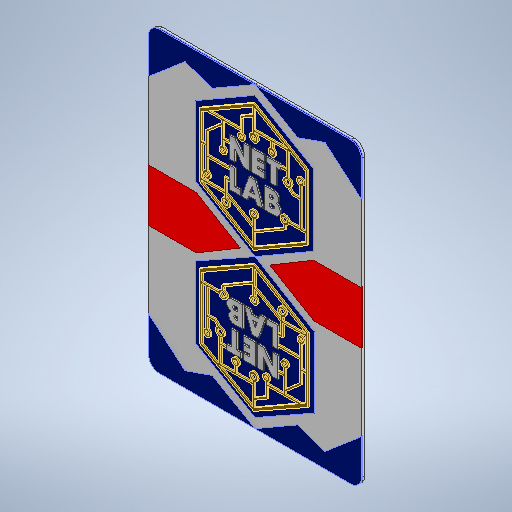
# Autodesk Inventor part: 4ofethernet
Saved by Autodesk Inventor 2025 (Build 290162010, 162A)
## iProperties
Created: 2024-07-12
Part Number: 4ofethernet
Material: Generic
Document SubType Name: Modeling
Designer: joshu
Density: 1 g/cm^3
Appearance: Default
Author: joshu
Autodesk Inventor part; units mm, degrees
(part 1 of 2)
ref_plane "YZ Plane" through (0, 0, 0) normal (1, 0, 0) x (0, 1, 0)
ref_plane "XZ Plane" through (0, 0, 0) normal (0, 1, 0) x (-1, 0, 0)
ref_plane "XY Plane" through (0, 0, 0) normal (0, 0, 1) x (1, 0, 0)
sketch "Sketch1" plane through (0, 0, 0) normal (0, 0, 1) x (1, 0, 0)
  line L0 (0, 0) -> (63.5, 0)
  line L1 (63.5, 0) -> (63.5, 88.9)
  line L2 (63.5, 88.9) -> (0, 88.9)
  line L3 (0, 88.9) -> (0, 0)
  line L4 (31.75, 44.45) -> (49.3079, 54.587)
  line L5 (49.3079, 54.587) -> (49.3079, 75.7826)
  line L6 (49.3079, 75.7826) -> (31.6801, 86.0828)
  line L7 (31.6801, 86.0828) -> (13.967, 75.8563)
  line L8 (13.967, 75.8563) -> (13.967, 55.04)
  line L9 (13.967, 55.04) -> (31.75, 44.45)
  line L10 (15.5263, 74.956) -> (31.6754, 84.2796)
  line L11 (31.6754, 84.2796) -> (47.7487, 74.8877)
  line L12 (47.7487, 74.8877) -> (47.7487, 55.4872)
  line L13 (47.7487, 55.4872) -> (31.7622, 46.2575)
  line L14 (31.7622, 46.2575) -> (15.5263, 55.9263)
  line L15 (15.5263, 55.9263) -> (15.5263, 74.956)
  line L16 (47.1273, 56.0392) -> (31.9379, 47.2671)
  line L17 (31.3664, 47.317) -> (16.2977, 56.192)
  line L18 (41.8086, 77.4972) -> (32.0418, 77.4972)
  line L19 (42.0908, 76.9257) -> (42.0908, 70.0939)
  line L20 (41.5193, 72.1376) -> (39.6994, 72.1376)
  line L21 (39.6994, 72.1376) -> (39.6994, 71.5661)
  line L22 (39.6994, 71.5661) -> (41.5193, 71.5661)
  arc A0 (31.465, 76.5861) -> (32.0365, 76.5861) centre (31.7507, 75.3324) ccw
  arc A1 (36.8763, 75.3571) -> (37.4478, 75.3571) centre (37.162, 74.2504) ccw
  circle A2 centre (37.162, 74.2504) radius 0.4762
  circle A3 centre (31.7507, 75.3324) radius 0.6191
  line L23 (45.9318, 69.8545) -> (45.9318, 58.9507)
  line L24 (45.3603, 66.7769) -> (43.3841, 66.7769)
  line L25 (43.1915, 66.2054) -> (45.3603, 66.2054)
  circle A4 centre (41.805, 68.7917) radius 0.762
  line L26 (43.1915, 66.2054) -> (41.9826, 67.4703)
  line L27 (43.3841, 66.7769) -> (42.5287, 67.6719)
  arc A5 (45.9318, 69.8545) -> (45.3603, 69.8545) centre (45.646, 70.9598) ccw
  circle A6 centre (45.646, 70.9598) radius 0.5715
  line L28 (40.6132, 56.5528) -> (40.6132, 57.4113)
  circle A7 centre (40.899, 58.665) radius 0.7144
  line L29 (32.0418, 83.1688) -> (32.0418, 77.4972)
  line L30 (32.0365, 76.9257) -> (32.0365, 76.5861)
  line L31 (32.0365, 76.9257) -> (36.8763, 76.9257)
  line L32 (36.8763, 75.3571) -> (36.8763, 76.9257)
  line L33 (37.4478, 76.9257) -> (37.4478, 75.3571)
  line L34 (37.4478, 76.9257) -> (41.5193, 76.9257)
  line L35 (42.0908, 76.9257) -> (42.7928, 76.9257)
  line L36 (32.0365, 83.1719) -> (41.8086, 77.4972)
  line L37 (42.7928, 76.9257) -> (47.1273, 74.4086)
  line L38 (41.5193, 70.0939) -> (41.5193, 71.5661)
  line L39 (41.5193, 72.1376) -> (41.5193, 76.9257)
  arc A8 (41.5193, 70.0939) -> (41.9826, 67.4703) centre (41.805, 68.7917) ccw
  arc A9 (42.5287, 67.6719) -> (42.0908, 70.0939) centre (41.805, 68.7917) ccw
  line L40 (45.3603, 58.9507) -> (45.3603, 66.2054)
  line L41 (45.3603, 66.7769) -> (45.3603, 69.8545)
  line L42 (47.1273, 58.9507) -> (45.9318, 58.9507)
  line L43 (45.3603, 58.9507) -> (42.1527, 58.9507)
  line L44 (42.1475, 58.3804) -> (47.1273, 58.3804)
  line L45 (41.1819, 57.4161) -> (41.1819, 56.2658)
  arc A10 (42.1527, 58.9507) -> (40.6132, 57.4113) centre (40.899, 58.665) ccw
  arc A11 (41.1819, 57.4161) -> (42.1475, 58.3804) centre (40.899, 58.665) ccw
  line L46 (47.1273, 74.4086) -> (47.1273, 58.9507)
  line L47 (47.1273, 58.3804) -> (47.1273, 56.0392)
  line L48 (27.6974, 78.6822) -> (27.6974, 79.0777)
  line L49 (28.2689, 78.6822) -> (31.465, 80.528)
  line L50 (27.6974, 79.0777) -> (31.465, 81.2535)
  line L51 (31.465, 76.5861) -> (31.465, 80.528)
  line L52 (31.465, 81.2535) -> (31.465, 83.1596)
  line L53 (31.9379, 51.4601) -> (40.6132, 56.5528)
  line L54 (31.9379, 50.8392) -> (41.1819, 56.2658)
  line L55 (16.2977, 57.1448) -> (22.9994, 57.1448)
  line L56 (22.9994, 56.5733) -> (16.2977, 56.5733)
  line L57 (16.2977, 56.5733) -> (16.2977, 57.1448)
  line L58 (22.9994, 60.9472) -> (23.5709, 60.9472)
  line L59 (22.9994, 60.9472) -> (24.4329, 60.9472)
  line L60 (24.4329, 60.9472) -> (24.4329, 60.3757)
  line L61 (24.4329, 60.3757) -> (23.5709, 60.3757)
  line L62 (22.9994, 60.3757) -> (22.9994, 60.9472)
  line L63 (23.5709, 56.4373) -> (31.3664, 51.9861)
  line L64 (31.3664, 52.5972) -> (23.5709, 57.0484)
  arc A12 (31.9379, 54.3552) -> (31.3664, 54.3552) centre (31.6521, 55.5111) ccw
  circle A13 centre (31.6521, 55.5111) radius 0.6191
  arc A14 (22.9994, 55.5805) -> (23.5709, 55.5805) centre (23.2852, 54.3309) ccw
  circle A15 centre (23.2852, 54.3309) radius 0.7144
  line L65 (23.5709, 60.3757) -> (23.5709, 57.0484)
  line L66 (23.5709, 56.4373) -> (23.5709, 55.5805)
  line L67 (22.9994, 55.5805) -> (22.9994, 56.5733)
  line L68 (22.9994, 57.1448) -> (22.9994, 60.9472)
  line L69 (31.3664, 54.3552) -> (31.3664, 52.5972)
  line L70 (31.3664, 51.9861) -> (31.3664, 47.317)
  line L71 (31.9379, 47.2671) -> (31.9379, 50.8392)
  line L72 (31.9379, 51.4601) -> (31.9379, 54.3552)
  arc A16 (27.6974, 74.6924) -> (28.2689, 74.6924) centre (27.9831, 73.6844) ccw
  circle A17 centre (27.9831, 73.6844) radius 0.4763
  line L73 (18.5492, 75.7007) -> (27.6974, 75.7007)
  line L74 (22.769, 70.6818) -> (24.4329, 70.6818)
  line L75 (24.4329, 70.6818) -> (24.4329, 70.1103)
  line L76 (24.4329, 70.1103) -> (22.769, 70.1103)
  line L77 (22.769, 70.1103) -> (22.769, 70.2009)
  line L78 (16.2977, 66.7769) -> (17.4065, 66.7769)
  line L79 (17.978, 66.7769) -> (17.978, 66.2054)
  line L80 (17.4065, 66.2054) -> (16.2977, 66.2054)
  line L81 (17.978, 63.9706) -> (24.4329, 63.9706)
  line L82 (24.4329, 63.9706) -> (24.4329, 63.3991)
  line L83 (24.4329, 63.3991) -> (17.978, 63.3991)
  line L84 (17.4065, 66.7769) -> (17.4065, 70.2549)
  line L85 (17.978, 70.0307) -> (17.978, 66.7769)
  line L86 (17.4065, 70.2549) -> (22.1975, 74.4365)
  line L87 (17.978, 70.0307) -> (22.1975, 73.7135)
  arc A18 (22.1975, 68.5281) -> (22.769, 68.5281) centre (22.4833, 67.4703) ccw
  circle A19 centre (22.4833, 67.4703) radius 0.5239
  line L88 (16.2977, 74.4004) -> (17.5596, 75.1292)
  line L89 (18.5492, 75.7007) -> (31.465, 83.1596)
  line L90 (27.6974, 75.1292) -> (22.769, 75.1292)
  line L91 (22.1975, 75.1292) -> (17.5596, 75.1292)
  line L92 (22.1975, 74.4365) -> (22.1975, 75.1292)
  line L93 (28.2689, 74.6924) -> (28.2689, 78.6822)
  line L94 (22.769, 75.1292) -> (22.769, 70.6818)
  line L95 (22.769, 70.1103) -> (22.769, 68.5281)
  line L96 (22.1975, 67.8875) -> (22.1975, 67.9094)
  line L97 (22.1975, 68.5281) -> (22.1975, 73.7135)
  line L98 (16.2977, 56.192) -> (16.2977, 66.2054)
  line L99 (16.2977, 66.7769) -> (16.2977, 74.4004)
  line L100 (17.978, 63.9706) -> (17.978, 66.2054)
  line L101 (27.6974, 78.6822) -> (27.6974, 75.7007)
  line L102 (27.6974, 75.1292) -> (27.6974, 74.6924)
  line L103 (24.4329, 66.1976) -> (26.1474, 66.1976)
  line L104 (26.1474, 66.1976) -> (26.1474, 69.7075)
  line L105 (26.1474, 72.4542) -> (24.4329, 72.4542)
  line L106 (24.4329, 72.4542) -> (24.4329, 66.1976)
  line L107 (28.7777, 72.4542) -> (30.4922, 72.4542)
  line L108 (30.4922, 72.4542) -> (30.4922, 66.1976)
  line L109 (30.4922, 66.1976) -> (28.7777, 66.1976)
  line L110 (28.7777, 68.9443) -> (28.7777, 72.4542)
  line L111 (28.7777, 66.1976) -> (26.1474, 69.7075)
  line L112 (26.1474, 72.4542) -> (28.7777, 68.9443)
  line L113 (31.2537, 72.4542) -> (32.9682, 72.4542)
  line L114 (32.9682, 66.1976) -> (31.2537, 66.1976)
  line L115 (31.2537, 66.1976) -> (31.2537, 72.4542)
  line L116 (31.2537, 72.4542) -> (34.8385, 72.4542)
  line L117 (34.8385, 72.4542) -> (34.8385, 70.7397)
  line L118 (34.8385, 70.7397) -> (32.9682, 70.7397)
  line L119 (31.2537, 70.7397) -> (31.2537, 72.4542)
  line L120 (32.9682, 70.0633) -> (34.8385, 70.0633)
  line L121 (34.8385, 70.0633) -> (34.8385, 68.5393)
  line L122 (34.8385, 68.5393) -> (32.9682, 68.5393)
  line L123 (31.2537, 68.5393) -> (31.2537, 70.0633)
  line L124 (31.2537, 66.1976) -> (34.8385, 66.1976)
  line L125 (34.8385, 66.1976) -> (34.8385, 67.9121)
  line L126 (34.8385, 67.9121) -> (32.9682, 67.9121)
  line L127 (31.2537, 67.9121) -> (31.2537, 66.1976)
  line L128 (32.9682, 70.7397) -> (32.9682, 70.0633)
  line L129 (32.9682, 68.5393) -> (32.9682, 67.9121)
  line L130 (39.6994, 72.4422) -> (35.4849, 72.4422)
  line L131 (35.4849, 72.4422) -> (35.4849, 70.9182)
  line L132 (39.6994, 70.9182) -> (39.6994, 72.4422)
  line L133 (38.4466, 70.9182) -> (38.4466, 66.1976)
  line L134 (38.4466, 66.1976) -> (36.7321, 66.1976)
  line L135 (36.7321, 66.1976) -> (36.7321, 70.9182)
  line L136 (36.7321, 70.9182) -> (36.8763, 70.9182)
  line L137 (35.4849, 70.9182) -> (36.7321, 70.9182)
  line L138 (38.4466, 70.9182) -> (39.6994, 70.9182)
  line L139 (24.4329, 64.6461) -> (26.1474, 64.6461)
  line L140 (26.1474, 64.6461) -> (26.1474, 59.9044)
  line L141 (26.1474, 58.3804) -> (24.4329, 58.3804)
  line L142 (24.4329, 58.3804) -> (24.4329, 64.6461)
  line L143 (24.4329, 58.3804) -> (27.8234, 58.3804)
  line L144 (27.8234, 58.3804) -> (27.8234, 59.9044)
  line L145 (27.8234, 59.9044) -> (26.1474, 59.9044)
  line L146 (24.4329, 59.9044) -> (24.4329, 58.3804)
  line L147 (28.1466, 58.3804) -> (29.8611, 58.3804)
  line L148 (29.8611, 58.3804) -> (30.3254, 59.5144)
  line L149 (30.3254, 59.5144) -> (32.2304, 59.5144)
  line L150 (30.3254, 64.6461) -> (32.2304, 64.6461)
  line L151 (28.1466, 58.3804) -> (30.3254, 64.6461)
  line L152 (32.728, 58.3804) -> (34.4425, 58.3804)
  line L153 (32.728, 58.3804) -> (32.2304, 59.5144)
  line L154 (34.4425, 58.3804) -> (32.2304, 64.6461)
  line L155 (30.6203, 60.8236) -> (31.9379, 60.8236)
  line L156 (31.9379, 60.8236) -> (31.2779, 62.4085)
  line L157 (31.2779, 62.4085) -> (30.6203, 60.8236)
  line L158 (34.9216, 58.3804) -> (34.9216, 64.6461)
  line L159 (34.9216, 64.6461) -> (37.8691, 64.6461)
  line L160 (34.9216, 58.3804) -> (37.8691, 58.3804)
  line L161 (36.5599, 59.8143) -> (36.5599, 60.939)
  line L162 (36.5599, 62.1736) -> (36.5599, 63.1944)
  line L163 (36.5599, 63.1944) -> (37.2133, 63.1944)
  line L164 (36.5599, 62.1736) -> (37.2133, 62.1736)
  arc A20 (37.2133, 62.1736) -> (37.2133, 63.1944) centre (37.055, 62.684) ccw
  line L165 (36.5599, 60.939) -> (37.4519, 60.939)
  line L166 (36.5599, 59.8143) -> (37.4396, 59.8143)
  arc A21 (37.4396, 59.8143) -> (37.4519, 60.939) centre (37.3959, 60.3772) ccw
  arc A22 (38.5631, 61.7817) -> (37.8691, 64.6461) centre (37.5266, 63.0469) ccw
  arc A23 (37.8691, 58.3804) -> (38.5631, 61.7817) centre (37.9604, 60.1332) ccw
  arc A24 (17.4065, 59.8724) -> (17.978, 59.8724) centre (17.6923, 58.815) ccw
  circle A25 centre (17.6923, 58.815) radius 0.5239
  line L167 (17.4065, 66.2054) -> (17.4065, 59.8724)
  line L168 (17.978, 59.8724) -> (17.978, 63.3991)
  line L169 (32.0418, 83.1688) -> (41.8086, 77.4972)
  line L170 (32.0418, 77.4972) -> (41.8086, 77.4972)
  line L171 (32.0418, 77.4972) -> (32.0418, 83.1688)
  line L172 (0, 44.45) -> (63.5, 44.45) construction
  line L173 (31.75, 88.9) -> (31.75, 0) construction
  line L174 (0, 52.2573) -> (14.2102, 52.2573)
  line L175 (14.2102, 52.2573) -> (27.3204, 44.45)
  line L176 (0, 36.6427) -> (14.2102, 36.6427)
  line L177 (14.2102, 36.6427) -> (27.3204, 44.45)
  line L178 (63.5, 52.2573) -> (49.2898, 52.2573)
  line L179 (49.2898, 52.2573) -> (36.1796, 44.45)
  line L180 (49.2898, 36.6427) -> (36.1796, 44.45)
  line L181 (63.5, 36.6427) -> (49.2898, 36.6427)
  line L182 (0, 75.0796) -> (10.8905, 84.3747)
  line L183 (10.8905, 84.3747) -> (18.9583, 81.5148)
  line L184 (18.9583, 81.5148) -> (31.75, 88.9)
  line L185 (63.5, 75.0796) -> (52.6095, 84.3747)
  line L186 (52.6095, 84.3747) -> (44.5417, 81.5148)
  line L187 (44.5417, 81.5148) -> (31.75, 88.9)
  line L188 (46.0393, 22.6946) -> (47.1481, 22.6946)
  line L189 (45.4678, 22.1231) -> (45.4678, 22.6946)
  line L190 (45.4678, 24.9294) -> (45.4678, 22.6946)
  line L191 (47.1481, 22.1231) -> (46.0393, 22.1231)
  line L192 (47.1481, 32.3267) -> (47.1481, 31.7552)
  line L193 (47.1481, 32.708) -> (47.1481, 22.6946)
  line L194 (47.1481, 31.7552) -> (40.4464, 31.7552)
  line L195 (40.4464, 32.3267) -> (47.1481, 32.3267)
  line L196 (45.4678, 29.0276) -> (45.4678, 25.5009)
  line L197 (46.0393, 22.6946) -> (46.0393, 29.0276)
  circle A26 centre (45.7535, 30.085) radius 0.5239
  arc A27 (46.0393, 29.0276) -> (45.4678, 29.0276) centre (45.7535, 30.085) ccw
  line L198 (20.6531, 11.9743) -> (16.3185, 14.4914)
  line L199 (21.355, 11.9743) -> (20.6531, 11.9743)
  line L200 (21.9265, 16.7624) -> (21.9265, 11.9743)
  line L201 (21.355, 11.9743) -> (21.355, 18.8061)
  line L202 (21.9265, 16.7624) -> (23.7464, 16.7624)
  line L203 (23.7464, 17.3339) -> (21.9265, 17.3339)
  line L204 (25.998, 11.9743) -> (21.9265, 11.9743)
  line L205 (26.5695, 13.5429) -> (26.5695, 11.9743)
  circle A28 centre (21.6408, 20.1083) radius 0.762
  circle A29 centre (26.2838, 14.6496) radius 0.4762
  arc A30 (26.5695, 13.5429) -> (25.998, 13.5429) centre (26.2838, 14.6496) ccw
  line L206 (31.4093, 11.9743) -> (26.5695, 11.9743)
  arc A31 (31.9808, 12.3139) -> (31.4093, 12.3139) centre (31.6951, 13.5676) ccw
  line L207 (25.998, 11.9743) -> (25.998, 13.5429)
  line L208 (45.4678, 24.9294) -> (39.013, 24.9294)
  line L209 (39.013, 25.5009) -> (45.4678, 25.5009)
  line L210 (39.013, 24.9294) -> (39.013, 25.5009)
  circle A32 centre (40.1606, 34.5691) radius 0.7144
  arc A33 (40.4464, 33.3195) -> (39.8749, 33.3195) centre (40.1606, 34.5691) ccw
  line L211 (39.8749, 32.4627) -> (39.8749, 33.3195)
  line L212 (40.4464, 33.3195) -> (40.4464, 32.3267)
  line L213 (39.013, 27.9528) -> (39.013, 28.5243)
  line L214 (39.8749, 28.5243) -> (39.8749, 31.8516)
  line L215 (39.013, 28.5243) -> (39.8749, 28.5243)
  line L216 (40.4464, 31.7552) -> (40.4464, 27.9528)
  line L217 (40.4464, 28.5243) -> (40.4464, 27.9528)
  line L218 (40.4464, 27.9528) -> (39.8749, 27.9528)
  line L219 (40.4464, 27.9528) -> (39.013, 27.9528)
  line L220 (33.5847, 30.5196) -> (33.1204, 29.3856)
  line L221 (35.6224, 28.9956) -> (37.2985, 28.9956)
  line L222 (35.2992, 30.5196) -> (33.5847, 30.5196)
  line L223 (39.013, 28.9956) -> (39.013, 30.5196)
  line L224 (35.2992, 30.5196) -> (33.1204, 24.2539)
  line L225 (46.0393, 18.6451) -> (41.2483, 14.4635)
  line L226 (45.4678, 18.8693) -> (41.2483, 15.1865)
  line L227 (40.6768, 18.7897) -> (40.6768, 20.3719)
  line L228 (41.2483, 21.0125) -> (41.2483, 20.9906)
  line L229 (41.2483, 20.3719) -> (41.2483, 15.1865)
  line L230 (40.6768, 13.7708) -> (40.6768, 18.2182)
  line L231 (41.2483, 14.4635) -> (41.2483, 13.7708)
  line L232 (41.2483, 13.7708) -> (45.8862, 13.7708)
  line L233 (47.1481, 22.1231) -> (47.1481, 14.4996)
  line L234 (47.1481, 14.4996) -> (45.8862, 13.7708)
  circle A34 centre (40.9626, 21.4297) radius 0.5239
  line L235 (32.8255, 28.0764) -> (31.5079, 28.0764)
  line L236 (32.1679, 26.4915) -> (32.8255, 28.0764)
  line L237 (31.5079, 28.0764) -> (32.1679, 26.4915)
  line L238 (33.1204, 29.3856) -> (31.2154, 29.3856)
  line L239 (35.6224, 30.5196) -> (35.6224, 28.9956)
  line L240 (37.2985, 24.2539) -> (37.2985, 28.9956)
  line L241 (37.2985, 30.5196) -> (39.013, 30.5196)
  line L242 (39.013, 30.5196) -> (39.013, 24.2539)
  line L243 (39.013, 30.5196) -> (35.6224, 30.5196)
  line L244 (39.013, 24.2539) -> (37.2985, 24.2539)
  line L245 (33.1204, 24.2539) -> (31.2154, 24.2539)
  line L246 (30.7178, 30.5196) -> (31.2154, 29.3856)
  line L247 (37.2985, 16.4458) -> (39.013, 16.4458)
  line L248 (40.6768, 18.2182) -> (39.013, 18.2182)
  line L249 (39.013, 18.7897) -> (40.6768, 18.7897)
  line L250 (40.6768, 18.7897) -> (40.6768, 18.6991)
  line L251 (39.013, 18.2182) -> (39.013, 18.7897)
  line L252 (46.0393, 22.1231) -> (46.0393, 18.6451)
  line L253 (45.4678, 18.8693) -> (45.4678, 22.1231)
  arc A35 (41.2483, 20.3719) -> (40.6768, 20.3719) centre (40.9626, 21.4297) ccw
  line L254 (39.013, 16.4458) -> (39.013, 22.7024)
  line L255 (39.013, 22.7024) -> (37.2985, 22.7024)
  line L256 (32.9536, 22.7024) -> (34.6681, 22.7024)
  line L257 (30.4777, 22.7024) -> (32.1922, 22.7024)
  line L258 (30.4777, 18.8367) -> (28.6073, 18.8367)
  line L259 (32.1922, 22.7024) -> (28.6073, 22.7024)
  line L260 (28.6073, 22.7024) -> (28.6073, 20.9879)
  line L261 (28.6073, 20.9879) -> (30.4777, 20.9879)
  line L262 (32.1922, 20.9879) -> (32.1922, 22.7024)
  line L263 (30.4777, 20.3607) -> (30.4777, 20.9879)
  line L264 (28.6073, 20.3607) -> (30.4777, 20.3607)
  line L265 (28.6073, 18.8367) -> (28.6073, 20.3607)
  line L266 (32.1922, 20.3607) -> (32.1922, 18.8367)
  line L267 (30.4777, 18.1603) -> (30.4777, 18.8367)
  line L268 (26.8859, 25.7056) -> (26.2325, 25.7056)
  line L269 (26.8859, 29.0857) -> (26.0062, 29.0857)
  line L270 (26.8859, 27.961) -> (25.9939, 27.961)
  line L271 (28.5242, 30.5196) -> (25.5767, 30.5196)
  line L272 (32.0794, 36.9139) -> (32.0794, 41.583)
  line L273 (31.5079, 41.6329) -> (31.5079, 38.0608)
  line L274 (26.8859, 26.7264) -> (26.8859, 25.7056)
  line L275 (28.5242, 24.2539) -> (25.5767, 24.2539)
  line L276 (29.0033, 30.5196) -> (31.2154, 24.2539)
  line L277 (30.7178, 30.5196) -> (29.0033, 30.5196)
  line L278 (26.8859, 26.7264) -> (26.2325, 26.7264)
  line L279 (28.5242, 30.5196) -> (28.5242, 24.2539)
  arc A36 (26.2325, 26.7264) -> (26.2325, 25.7056) centre (26.3908, 26.216) ccw
  line L280 (26.8859, 29.0857) -> (26.8859, 27.961)
  arc A37 (26.0062, 29.0857) -> (25.9939, 27.961) centre (26.0499, 28.5228) ccw
  arc A38 (24.8827, 27.1183) -> (25.5767, 24.2539) centre (25.9192, 25.8531) ccw
  arc A39 (25.5767, 30.5196) -> (24.8827, 27.1183) centre (25.4854, 28.7668) ccw
  line L281 (23.7464, 16.7624) -> (23.7464, 17.3339)
  line L282 (24.9992, 22.7024) -> (26.7137, 22.7024)
  line L283 (27.961, 17.9818) -> (26.7137, 17.9818)
  line L284 (26.7137, 22.7024) -> (26.7137, 17.9818)
  line L285 (26.7137, 17.9818) -> (26.5695, 17.9818)
  line L286 (24.9992, 17.9818) -> (24.9992, 22.7024)
  line L287 (24.9992, 17.9818) -> (23.7464, 17.9818)
  line L288 (27.961, 16.4578) -> (27.961, 17.9818)
  line L289 (23.7464, 16.4578) -> (27.961, 16.4578)
  line L290 (23.7464, 17.9818) -> (23.7464, 16.4578)
  line L291 (31.75, 44.45) -> (14.1379, 34.5158)
  line L292 (15.6972, 33.6051) -> (31.7276, 42.6471)
  line L293 (16.3185, 32.8608) -> (31.5079, 41.6329)
  line L294 (31.5079, 37.4399) -> (22.8326, 32.3472)
  line L295 (31.5079, 38.0608) -> (22.2639, 32.6342)
  line L296 (31.5079, 37.4399) -> (31.5079, 34.5448)
  line L297 (35.7484, 10.2178) -> (35.7484, 9.8223)
  line L298 (35.1769, 10.2178) -> (31.9808, 8.372)
  line L299 (35.7484, 9.8223) -> (31.9808, 7.6465)
  line L300 (31.9808, 12.3139) -> (31.9808, 8.372)
  line L301 (31.9808, 7.6465) -> (31.9808, 5.7404)
  circle A40 centre (35.4627, 15.2156) radius 0.4763
  arc A41 (35.7484, 14.2076) -> (35.1769, 14.2076) centre (35.4627, 15.2156) ccw
  line L302 (35.7484, 13.7708) -> (35.7484, 14.2076)
  line L303 (35.7484, 13.7708) -> (40.6768, 13.7708)
  line L304 (44.8966, 13.1993) -> (35.7484, 13.1993)
  line L305 (35.1769, 14.2076) -> (35.1769, 10.2178)
  line L306 (35.7484, 10.2178) -> (35.7484, 13.1993)
  line L307 (44.8966, 13.1993) -> (31.9808, 5.7404)
  line L308 (31.4093, 11.9743) -> (31.4093, 12.3139)
  line L309 (47.9195, 13.7706) -> (31.7623, 4.657)
  circle A42 centre (31.6951, 13.5676) radius 0.6191
  line L310 (31.7499, 2.8598) -> (49.4788, 12.8599)
  line L311 (47.9195, 32.9751) -> (47.9195, 13.7706)
  line L312 (49.4788, 12.8599) -> (49.4788, 33.86)
  circle A43 centre (31.7937, 33.3889) radius 0.6191
  line L313 (32.0794, 41.583) -> (47.1481, 32.708)
  line L314 (49.4788, 33.86) -> (31.75, 44.45)
  line L315 (31.7276, 42.6471) -> (47.9195, 32.9751)
  line L316 (32.0794, 36.3028) -> (39.8749, 31.8516)
  line L317 (39.8749, 32.4627) -> (32.0794, 36.9139)
  line L318 (32.0794, 34.5448) -> (32.0794, 36.3028)
  arc A44 (31.5079, 34.5448) -> (32.0794, 34.5448) centre (31.7937, 33.3889) ccw
  circle A45 centre (17.7998, 17.9402) radius 0.5715
  line L319 (18.0855, 22.1231) -> (20.0617, 22.1231)
  line L320 (20.2543, 22.6946) -> (18.0855, 22.6946)
  line L321 (22.8326, 32.3472) -> (22.8326, 31.4887)
  circle A46 centre (22.5468, 30.235) radius 0.7144
  line L322 (21.2984, 30.5196) -> (16.3185, 30.5196)
  line L323 (22.2639, 31.4839) -> (22.2639, 32.6342)
  arc A47 (21.2931, 29.9493) -> (22.8326, 31.4887) centre (22.5468, 30.235) ccw
  arc A48 (22.2639, 31.4839) -> (21.2984, 30.5196) centre (22.5468, 30.235) ccw
  line L324 (16.3185, 30.5196) -> (16.3185, 32.8608)
  line L325 (14.1379, 34.5158) -> (14.1379, 13.1174)
  line L326 (15.6972, 14.0137) -> (15.6972, 33.6051)
  line L327 (17.514, 19.0455) -> (17.514, 29.9493)
  line L328 (20.2543, 22.6946) -> (21.4633, 21.4297)
  line L329 (20.0617, 22.1231) -> (20.9171, 21.2281)
  arc A49 (17.514, 19.0455) -> (18.0855, 19.0455) centre (17.7998, 17.9402) ccw
  line L330 (21.9265, 18.8061) -> (21.9265, 17.3339)
  arc A50 (20.9171, 21.2281) -> (21.355, 18.8061) centre (21.6408, 20.1083) ccw
  line L331 (18.0855, 22.1231) -> (18.0855, 19.0455)
  line L332 (16.3185, 14.4914) -> (16.3185, 29.9493)
  line L333 (16.3185, 29.9493) -> (17.514, 29.9493)
  line L334 (18.0855, 29.9493) -> (18.0855, 22.6946)
  line L335 (18.0855, 29.9493) -> (21.2931, 29.9493)
  arc A51 (21.9265, 18.8061) -> (21.4633, 21.4297) centre (21.6408, 20.1083) ccw
  line L336 (14.1379, 13.1174) -> (31.7499, 2.8598)
  line L337 (31.7623, 4.657) -> (15.6972, 14.0137)
  line L338 (21.6372, 11.4028) -> (31.404, 11.4028)
  line L339 (31.404, 11.4028) -> (31.404, 5.7312)
  line L340 (31.404, 5.7312) -> (21.6372, 11.4028)
  line L341 (37.2985, 22.7024) -> (37.2985, 19.1925)
  line L342 (34.6681, 16.4458) -> (32.9536, 16.4458)
  line L343 (32.9536, 16.4458) -> (32.9536, 22.7024)
  line L344 (34.6681, 22.7024) -> (37.2985, 19.1925)
  line L345 (28.6073, 18.1603) -> (30.4777, 18.1603)
  line L346 (32.1922, 16.4458) -> (28.6073, 16.4458)
  line L347 (28.6073, 16.4458) -> (28.6073, 18.1603)
  line L348 (32.1922, 22.7024) -> (32.1922, 16.4458)
  line L349 (32.1922, 16.4458) -> (30.4777, 16.4458)
  line L350 (34.6681, 19.9557) -> (34.6681, 16.4458)
  line L351 (37.2985, 16.4458) -> (34.6681, 19.9557)
  line L352 (32.1922, 18.1603) -> (32.1922, 16.4458)
  line L353 (0, 13.8204) -> (10.8905, 4.5253)
  line L354 (10.8905, 4.5253) -> (18.9583, 7.3852)
  line L355 (18.9583, 7.3852) -> (31.75, 0)
  line L356 (63.5, 13.8204) -> (52.6095, 4.5253)
  line L357 (52.6095, 4.5253) -> (44.5417, 7.3852)
  line L358 (44.5417, 7.3852) -> (31.75, 0)
  point P0 (31.9379, 47.317)
  point P1 (31.7229, 65.2666)
  point P2 (31.7229, 23.6334)
  point P3 (31.7229, 23.6334)
  point P4 (31.9379, 5.6837)
  point P5 (63.5, 75.0796)
  dimension "d0" = 63.5
  dimension "d1" = 88.9
  dimension "d43" = 44.45
  dimension "d99" = 120
  constraints: 718 end point, 170 parallel, 64 point on circle, 50 centre point, 42 perpendicular, 36 horizontal, 21 point on line, 20 coincident, 19 symmetric about line, 7 collinear, 5 midpoint, 4 vertical, 17 other
  measures "d0" distance of L2.end L1.end
  measures "d1" distance of L1.end L0.end
  measures "d43" distance between parallel lines of L172 L2
  measures "d99" angle of L357 L356
extrude "Extrusion1" add sketch "Sketch1" along normal blind 0.4 contours L3 L353 L354 L355 L0 | L358 L357 L356 L1 L0 | L3 L2 L184 L183 L182 | L185 L186 L187 L2 L1 | L9 L8 L7 L6 L5 L4 | L314 L312 L310 L336 L325 L291 | L10 L11 L12 L13 L14 L15 | L16 L71 L54 L45 A11 L44 L47 | L17 L98 L56 L67 A14 L66 L63 L70 | L18 L29 L36 | L35 L37 L46 L42 L23 A5 L41 L24 L27 A9 L19 | L20 L132 L130 L131 L137 L135 L134 L133 L138 L22 L38 A8 L26 L25 L40 L43 A10 L28 L53 L72 A12 L69 L64 L65 L61 L142 L141 L143 L144 L145 L140 L139 L81 L100 L79 L85 L87 L97 A18 L95 L76 L106 L103 L104 L111 L109 L108 L107 L110 L112 L105 L74 L94 L90 L102 A16 L93 L49 L51 A0 L30 L31 L32 A1 L33 L34 L39 | L21 L132 L138 L133 L134 L135 L137 L131 L130 | L106 L105 L112 L110 L107 L108 L109 L111 L104 L103 L75 | L60 L142 L82 L139 L140 L145 L144 L143 L141 | L59 L58 L62 L68 L55 L98 L80 L167 A24 L168 L83 L142 | A2 | A3 | A4 | A6 | A7 | L101 L73 L89 L52 L50 L48 | A13 | A15 | A17 | L99 L88 L91 L92 L86 L84 L78 | A19 | L113 L116 L117 L118 L128 L120 L121 L122 L129 L126 L125 L124 L114 L115 | L151 L150 L154 L152 L153 L149 L148 L147 | L157 L156 L155 | L158 L159 A22 A23 L160 | L161 L165 A21 L166 | L162 L163 A20 L164 | A25 | L197 A27 L196 L209 L242 L219 L218 L216 L194 L193 L188 | L210 L242 L244 L240 L221 L239 L243 L241 L223 L213 | L208 L190 L189 L253 L226 L229 A35 L227 L249 L254 L255 L341 L344 L256 L343 L342 L350 L351 L247 L248 L230 L303 L302 A41 L305 L298 L300 A31 L308 L206 L205 A30 L207 L204 L200 L202 L290 L289 L288 L283 L284 L282 L286 L287 L203 L330 A51 L328 L320 L334 L335 A47 L321 L294 L296 A44 L318 L316 L214 L215 L242 L223 L241 L243 L239 L221 L240 L244 | L251 L254 L247 L351 L350 L342 L343 L256 L344 L341 L255 | L290 L287 L286 L282 L284 L283 L288 L289 L281 | L233 L234 L232 L231 L225 L252 L191 | L193 L195 L212 A33 L211 L317 L272 L313 | A26 | L198 L332 L333 L327 A49 L331 L319 L329 A50 L201 L199 | A28 | A29 | A32 | L222 L224 L245 L276 L277 L246 L238 L220 | A34 | L236 L237 L235 | L257 L262 L348 L266 L346 L347 L345 L267 L258 L265 L264 L263 L261 L260 L259 | L268 A36 L278 L274 | L280 L270 A37 L269 | L279 L275 A38 A39 L271 | L273 L295 L323 A48 L322 L324 L293 | L292 L315 L311 L309 L337 L326 | L306 L304 L307 L301 L299 L297 | A40 | A42 | A43 | A45 | A46 | L338 L339 L340
extrude "Extrusion12" add sketch "Sketch1" along normal blind 0.4 separate body contours L3 L174 L175 L177 L176 | L181 L180 L179 L178 L1
extrude "Extrusion13" add sketch "Sketch1" along normal blind 0.4 separate body contours L355 L354 L353 L3 L176 L177 L175 L174 L182 L183 L184 L187 L186 L185 L1 L178 L179 L180 L181 L356 L357 L358
extrude "Extrusion14" add sketch "Sketch1" against normal blind 0.4 contours L21 L132 L138 L133 L134 L135 L137 L131 L130 | L106 L105 L112 L110 L107 L108 L109 L111 L104 L103 L75 | L60 L142 L82 L139 L140 L145 L144 L143 L141 | L113 L116 L117 L118 L128 L120 L121 L122 L129 L126 L125 L124 L114 L115 | L151 L150 L154 L152 L153 L149 L148 L147 | L158 L159 A22 A23 L160 | L210 L242 L244 L240 L221 L239 L243 L241 L223 L213 | L251 L254 L247 L351 L350 L342 L343 L256 L344 L341 L255 | L290 L287 L286 L282 L284 L283 L288 L289 L281 | L222 L224 L245 L276 L277 L246 L238 L220 | L257 L262 L348 L266 L346 L347 L345 L267 L258 L265 L264 L263 L261 L260 L259 | L279 L275 A38 A39 L271 bodies 3
extrude "Extrusion15" add sketch "Sketch1" against normal blind 0.4 separate body contours L10 L11 L12 L13 L14 L15 | L292 L315 L311 L309 L337 L326
pattern_linear "Rectangular Pattern1" count 2 spacing 0.8 along (0, 0, 1) of "Extrusion15" bodies 4
pattern_linear "Rectangular Pattern2" count 2 spacing 0.8 along (0, 0, 1) of "Extrusion14" bodies 3
extrude "Extrusion16" cut sketch "Sketch1" against normal blind 0.4 contours L9 L8 L7 L6 L5 L4 | L314 L312 L310 L336 L325 L291 | L10 L11 L12 L13 L14 L15 | L16 L71 L54 L45 A11 L44 L47 | L17 L98 L56 L67 A14 L66 L63 L70 | L18 L29 L36 | L35 L37 L46 L42 L23 A5 L41 L24 L27 A9 L19 | L20 L132 L130 L131 L137 L135 L134 L133 L138 L22 L38 A8 L26 L25 L40 L43 A10 L28 L53 L72 A12 L69 L64 L65 L61 L142 L141 L143 L144 L145 L140 L139 L81 L100 L79 L85 L87 L97 A18 L95 L76 L106 L103 L104 L111 L109 L108 L107 L110 L112 L105 L74 L94 L90 L102 A16 L93 L49 L51 A0 L30 L31 L32 A1 L33 L34 L39 | L21 L132 L138 L133 L134 L135 L137 L131 L130 | L106 L105 L112 L110 L107 L108 L109 L111 L104 L103 L75 | L60 L142 L82 L139 L140 L145 L144 L143 L141 | L59 L58 L62 L68 L55 L98 L80 L167 A24 L168 L83 L142 | A2 | A3 | A4 | A6 | A7 | L101 L73 L89 L52 L50 L48 | A13 | A15 | A17 | L99 L88 L91 L92 L86 L84 L78 | A19 | L113 L116 L117 L118 L128 L120 L121 L122 L129 L126 L125 L124 L114 L115 | L151 L150 L154 L152 L153 L149 L148 L147 | L157 L156 L155 | L158 L159 A22 A23 L160 | L161 L165 A21 L166 | L162 L163 A20 L164 | A25 | L197 A27 L196 L209 L242 L219 L218 L216 L194 L193 L188 | L210 L242 L244 L240 L221 L239 L243 L241 L223 L213 | L208 L190 L189 L253 L226 L229 A35 L227 L249 L254 L255 L341 L344 L256 L343 L342 L350 L351 L247 L248 L230 L303 L302 A41 L305 L298 L300 A31 L308 L206 L205 A30 L207 L204 L200 L202 L290 L289 L288 L283 L284 L282 L286 L287 L203 L330 A51 L328 L320 L334 L335 A47 L321 L294 L296 A44 L318 L316 L214 L215 L242 L223 L241 L243 L239 L221 L240 L244 | L251 L254 L247 L351 L350 L342 L343 L256 L344 L341 L255 | L290 L287 L286 L282 L284 L283 L288 L289 L281 | L233 L234 L232 L231 L225 L252 L191 | L193 L195 L212 A33 L211 L317 L272 L313 | A26 | L198 L332 L333 L327 A49 L331 L319 L329 A50 L201 L199 | A28 | A29 | A32 | L222 L224 L245 L276 L277 L246 L238 L220 | A34 | L236 L237 L235 | L257 L262 L348 L266 L346 L347 L345 L267 L258 L265 L264 L263 L261 L260 L259 | L268 A36 L278 L274 | L280 L270 A37 L269 | L279 L275 A38 A39 L271 | L273 L295 L323 A48 L322 L324 L293 | L292 L315 L311 L309 L337 L326 | L306 L304 L307 L301 L299 L297 | A40 | A42 | A43 | A45 | A46 | L338 L339 L340 bodies 3
extrude "Extrusion17" cut sketch "Sketch1" against normal blind 25.4 contours L9 L8 L7 L6 L5 L4 | L314 L312 L310 L336 L325 L291 | L10 L11 L12 L13 L14 L15 | L16 L71 L54 L45 A11 L44 L47 | L17 L98 L56 L67 A14 L66 L63 L70 | L18 L29 L36 | L35 L37 L46 L42 L23 A5 L41 L24 L27 A9 L19 | L20 L132 L130 L131 L137 L135 L134 L133 L138 L22 L38 A8 L26 L25 L40 L43 A10 L28 L53 L72 A12 L69 L64 L65 L61 L142 L141 L143 L144 L145 L140 L139 L81 L100 L79 L85 L87 L97 A18 L95 L76 L106 L103 L104 L111 L109 L108 L107 L110 L112 L105 L74 L94 L90 L102 A16 L93 L49 L51 A0 L30 L31 L32 A1 L33 L34 L39 | L21 L132 L138 L133 L134 L135 L137 L131 L130 | L106 L105 L112 L110 L107 L108 L109 L111 L104 L103 L75 | L60 L142 L82 L139 L140 L145 L144 L143 L141 | L59 L58 L62 L68 L55 L98 L80 L167 A24 L168 L83 L142 | A2 | A3 | A4 | A6 | A7 | L101 L73 L89 L52 L50 L48 | A13 | A15 | A17 | L99 L88 L91 L92 L86 L84 L78 | A19 | L113 L116 L117 L118 L128 L120 L121 L122 L129 L126 L125 L124 L114 L115 | L151 L150 L154 L152 L153 L149 L148 L147 | L157 L156 L155 | L158 L159 A22 A23 L160 | L161 L165 A21 L166 | L162 L163 A20 L164 | A25 | L197 A27 L196 L209 L242 L219 L218 L216 L194 L193 L188 | L210 L242 L244 L240 L221 L239 L243 L241 L223 L213 | L208 L190 L189 L253 L226 L229 A35 L227 L249 L254 L255 L341 L344 L256 L343 L342 L350 L351 L247 L248 L230 L303 L302 A41 L305 L298 L300 A31 L308 L206 L205 A30 L207 L204 L200 L202 L290 L289 L288 L283 L284 L282 L286 L287 L203 L330 A51 L328 L320 L334 L335 A47 L321 L294 L296 A44 L318 L316 L214 L215 L242 L223 L241 L243 L239 L221 L240 L244 | L251 L254 L247 L351 L350 L342 L343 L256 L344 L341 L255 | L290 L287 L286 L282 L284 L283 L288 L289 L281 | L233 L234 L232 L231 L225 L252 L191 | L193 L195 L212 A33 L211 L317 L272 L313 | A26 | L198 L332 L333 L327 A49 L331 L319 L329 A50 L201 L199 | A28 | A29 | A32 | L222 L224 L245 L276 L277 L246 L238 L220 | A34 | L236 L237 L235 | L257 L262 L348 L266 L346 L347 L345 L267 L258 L265 L264 L263 L261 L260 L259 | L268 A36 L278 L274 | L280 L270 A37 L269 | L279 L275 A38 A39 L271 | L273 L295 L323 A48 L322 L324 L293 | L292 L315 L311 L309 L337 L326 | L306 L304 L307 L301 L299 L297 | A40 | A42 | A43 | A45 | A46 | L338 L339 L340 bodies 4
sketch "Sketch14" plane through (0, 0, 0) normal (0, 0, -1) x (-1, 0, 0)
  line L0 (-63.5, 75.0796) -> (-63.5, 88.9) projected
  line L1 (0, 0) -> (-63.5, 0)
  line L2 (-63.5, 0) -> (-63.5, 88.9)
  line L3 (-63.5, 88.9) -> (0, 88.9)
  line L4 (0, 88.9) -> (0, 0)
  line L5 (-62.5, 1) -> (-1, 1)
  line L6 (-1, 1) -> (-1, 87.9)
  line L7 (-1, 87.9) -> (-62.5, 87.9)
  line L8 (-62.5, 87.9) -> (-62.5, 1)
  dimension "d90" = 1
  constraints: 16 end point, 4 parallel, 2 perpendicular, 1 horizontal, 3 other
  measures "d90" distance between parallel lines of L1 L5
extrude "Extrusion18" add sketch "Sketch14" along normal blind 0.2 separate body contours L8 L7 L6 L5
sketch "Sketch16" plane through (0, 0, 0) normal (0, 0, -1) x (-1, 0, 0)
  line L0 (-1, 1) -> (-1, 87.9) projected
  line L1 (-1, 87.9) -> (-62.5, 87.9) projected
  line L2 (-62.5, 87.9) -> (-62.5, 1) projected
  line L3 (-62.5, 1) -> (-1, 1) projected
  line L4 (0, 88.9) -> (0, 75.0796) projected
  line L5 (-31.75, 0) -> (-63.5, 0) projected
  line L6 (0, 88.9) -> (-63.5, 88.9)
  line L7 (-63.5, 88.9) -> (-63.5, 0)
  line L8 (-63.5, 0) -> (0, 0)
  line L9 (0, 0) -> (0, 88.9)
  constraints: 8 end point, 2 parallel, 1 horizontal, 1 perpendicular
extrude "Extrusion19" add sketch "Sketch16" along normal blind 0.2 bodies 3
sketch "Sketch17" plane through (0, 0, -0.2) normal (0, 0, -1) x (-1, 0, 0)
  line L0 (-63.5, 88.9) -> (-63.5, 0)
  line L1 (-63.5, 0) -> (0, 0)
  line L2 (0, 0) -> (0, 88.9)
  line L3 (0, 88.9) -> (-63.5, 88.9)
  line L4 (-62.5, 1) -> (-62.5, 87.9) construction
  line L5 (-1, 87.9) -> (-1, 1) construction
  line L6 (-62.5, 87.9) -> (-1, 87.9) projected
  line L7 (-1, 1) -> (-62.5, 1) projected
  line L8 (-40.1035, 96.9031) -> (-44.0256, 96.9031)
  line L9 (-44.0256, 96.9031) -> (-44.0256, 100.329)
  line L10 (-40.1035, 100.329) -> (-40.1035, 96.9031)
  line L11 (-43.1826, 97.7462) -> (-40.9465, 97.7462)
  line L12 (-40.9465, 97.7462) -> (-40.9465, 99.4859)
  line L13 (-40.9465, 99.4859) -> (-43.1826, 99.4859)
  line L14 (-43.1826, 99.4859) -> (-43.1826, 97.7462)
  line L15 (-40.8743, 102.5798) -> (-40.8743, 106.0056)
  line L16 (-40.8743, 106.0056) -> (-36.9522, 106.0056)
  line L17 (-36.9522, 106.0056) -> (-36.9522, 102.5798)
  line L18 (-40.0313, 103.4228) -> (-37.7953, 103.4228)
  line L19 (-37.7953, 103.4228) -> (-37.7953, 105.1626)
  line L20 (-37.7953, 105.1626) -> (-40.0313, 105.1626)
  line L21 (-40.0313, 105.1626) -> (-40.0313, 103.4228)
  line L22 (-46.961, 102.5567) -> (-46.961, 105.9825)
  line L23 (-46.961, 105.9825) -> (-43.039, 105.9825)
  line L24 (-43.039, 105.9825) -> (-43.039, 102.5567)
  line L25 (-46.118, 103.3997) -> (-43.882, 103.3997)
  line L26 (-43.882, 103.3997) -> (-43.882, 105.1395)
  line L27 (-43.882, 105.1395) -> (-46.118, 105.1395)
  line L28 (-46.118, 105.1395) -> (-46.118, 103.3997)
  line L29 (-46.8396, 101.057) -> (-46.8396, 101.7849)
  line L30 (-36.4128, 101.7849) -> (-36.4128, 101.057)
  line L31 (-42.4983, 100.329) -> (-42.4983, 101.057)
  line L32 (-41.6149, 101.057) -> (-41.6149, 100.329)
  line L33 (-44.0256, 100.329) -> (-42.4983, 100.329)
  line L34 (-41.6149, 100.329) -> (-40.1035, 100.329)
  line L35 (-36.4128, 101.057) -> (-41.6149, 101.057)
  line L36 (-42.4983, 101.057) -> (-46.8396, 101.057)
  line L37 (-39.4306, 101.7849) -> (-39.4306, 102.5798)
  line L38 (-38.6183, 102.5798) -> (-38.6183, 101.7849)
  line L39 (-45.6001, 101.7849) -> (-45.6001, 102.5567)
  line L40 (-44.6689, 102.5567) -> (-44.6689, 101.7849)
  line L41 (-36.9522, 102.5798) -> (-38.6183, 102.5798)
  line L42 (-39.4306, 102.5798) -> (-40.8743, 102.5798)
  line L43 (-38.6183, 101.7849) -> (-36.4128, 101.7849)
  line L44 (-43.039, 102.5567) -> (-44.6689, 102.5567)
  line L45 (-45.6001, 102.5567) -> (-46.961, 102.5567)
  line L46 (-46.8396, 101.7849) -> (-45.6001, 101.7849)
  line L47 (-44.6689, 101.7849) -> (-39.4306, 101.7849)
  line L48 (-42.893, 81.5577) -> (-37.6636, 81.5577)
  line L49 (-37.6636, 81.5577) -> (-37.6636, 76.9899)
  line L50 (-42.893, 76.9899) -> (-42.893, 81.5577)
  line L51 (-38.7876, 80.4336) -> (-41.769, 80.4336)
  line L52 (-41.769, 80.4336) -> (-41.769, 78.114)
  line L53 (-41.769, 78.114) -> (-38.7876, 78.114)
  line L54 (-38.7876, 78.114) -> (-38.7876, 80.4336)
  line L55 (-41.8653, 69.4211) -> (-47.0948, 69.4211)
  line L56 (-45.9707, 70.5451) -> (-42.9894, 70.5451)
  line L57 (-42.9894, 72.8648) -> (-45.9707, 72.8648)
  line L58 (-45.9707, 72.8648) -> (-45.9707, 70.5451)
  line L59 (-42.9894, 70.5451) -> (-42.9894, 72.8648)
  line L60 (-41.8653, 73.9888) -> (-41.8653, 69.4211)
  line L61 (-47.0948, 69.4211) -> (-47.0948, 73.9888)
  line L62 (-33.7497, 69.4518) -> (-38.9791, 69.4518)
  line L63 (-37.8551, 70.5759) -> (-34.8737, 70.5759)
  line L64 (-34.8737, 72.8956) -> (-37.8551, 72.8956)
  line L65 (-37.8551, 72.8956) -> (-37.8551, 70.5759)
  line L66 (-34.8737, 70.5759) -> (-34.8737, 72.8956)
  line L67 (-33.7497, 74.0196) -> (-33.7497, 69.4518)
  line L68 (-38.9791, 69.4518) -> (-38.9791, 74.0196)
  line L69 (-33.9116, 76.0192) -> (-33.9116, 75.0487)
  line L70 (-47.814, 75.0487) -> (-47.814, 76.0192)
  line L71 (-39.7, 76.9899) -> (-39.7, 76.0192)
  line L72 (-40.8779, 76.0192) -> (-40.8779, 76.9899)
  line L73 (-37.6636, 76.9899) -> (-39.7, 76.9899)
  line L74 (-40.8779, 76.9899) -> (-42.893, 76.9899)
  line L75 (-47.814, 76.0192) -> (-40.8779, 76.0192)
  line L76 (-39.7, 76.0192) -> (-33.9116, 76.0192)
  line L77 (-43.7903, 75.0487) -> (-43.7903, 73.9888)
  line L78 (-44.8734, 73.9888) -> (-44.8734, 75.0487)
  line L79 (-35.5643, 75.0487) -> (-35.5643, 74.0196)
  line L80 (-36.8058, 74.0196) -> (-36.8058, 75.0487)
  line L81 (-47.0948, 73.9888) -> (-44.8734, 73.9888)
  line L82 (-43.7903, 73.9888) -> (-41.8653, 73.9888)
  line L83 (-44.8734, 75.0487) -> (-47.814, 75.0487)
  line L84 (-38.9791, 74.0196) -> (-36.8058, 74.0196)
  line L85 (-35.5643, 74.0196) -> (-33.7497, 74.0196)
  line L86 (-33.9116, 75.0487) -> (-35.5643, 75.0487)
  line L87 (-36.8058, 75.0487) -> (-43.7903, 75.0487)
  line L88 (-55.4792, 73.4136) -> (-51.5572, 73.4136)
  line L89 (-51.5572, 73.4136) -> (-51.5572, 69.9878)
  line L90 (-55.4792, 69.9878) -> (-55.4792, 73.4136)
  line L91 (-52.4002, 72.5706) -> (-54.6362, 72.5706)
  line L92 (-54.6362, 72.5706) -> (-54.6362, 70.8308)
  line L93 (-54.6362, 70.8308) -> (-52.4002, 70.8308)
  line L94 (-52.4002, 70.8308) -> (-52.4002, 72.5706)
  line L95 (-54.7084, 64.3111) -> (-58.6305, 64.3111)
  line L96 (-57.7875, 65.1542) -> (-55.5515, 65.1542)
  line L97 (-55.5515, 66.8939) -> (-57.7875, 66.8939)
  line L98 (-57.7875, 66.8939) -> (-57.7875, 65.1542)
  line L99 (-55.5515, 65.1542) -> (-55.5515, 66.8939)
  line L100 (-54.7084, 67.737) -> (-54.7084, 64.3111)
  line L101 (-58.6305, 64.3111) -> (-58.6305, 67.737)
  line L102 (-48.6217, 64.3342) -> (-52.5438, 64.3342)
  line L103 (-51.7008, 65.1772) -> (-49.4647, 65.1772)
  line L104 (-49.4647, 66.917) -> (-51.7008, 66.917)
  line L105 (-51.7008, 66.917) -> (-51.7008, 65.1772)
  line L106 (-49.4647, 65.1772) -> (-49.4647, 66.917)
  line L107 (-48.6217, 67.76) -> (-48.6217, 64.3342)
  line L108 (-52.5438, 64.3342) -> (-52.5438, 67.76)
  line L109 (-48.7432, 69.2598) -> (-48.7432, 68.5318)
  line L110 (-59.17, 68.5318) -> (-59.17, 69.2598)
  line L111 (-53.0845, 69.9878) -> (-53.0845, 69.2598)
  line L112 (-53.9679, 69.2598) -> (-53.9679, 69.9878)
  line L113 (-51.5572, 69.9878) -> (-53.0845, 69.9878)
  line L114 (-53.9679, 69.9878) -> (-55.4792, 69.9878)
  line L115 (-59.17, 69.2598) -> (-53.9679, 69.2598)
  line L116 (-53.0845, 69.2598) -> (-48.7432, 69.2598)
  line L117 (-56.1521, 68.5318) -> (-56.1521, 67.737)
  line L118 (-56.9645, 67.737) -> (-56.9645, 68.5318)
  line L119 (-49.9827, 68.5318) -> (-49.9827, 67.76)
  line L120 (-50.9138, 67.76) -> (-50.9138, 68.5318)
  line L121 (-58.6305, 67.737) -> (-56.9645, 67.737)
  line L122 (-56.1521, 67.737) -> (-54.7084, 67.737)
  line L123 (-56.9645, 68.5318) -> (-59.17, 68.5318)
  line L124 (-52.5438, 67.76) -> (-50.9138, 67.76)
  line L125 (-49.9827, 67.76) -> (-48.6217, 67.76)
  line L126 (-48.7432, 68.5318) -> (-49.9827, 68.5318)
  line L127 (-50.9138, 68.5318) -> (-56.1521, 68.5318)
  line L128 (-8.0208, 15.4864) -> (-11.9428, 15.4864)
  line L129 (-11.9428, 15.4864) -> (-11.9428, 18.9122)
  line L130 (-8.0208, 18.9122) -> (-8.0208, 15.4864)
  line L131 (-11.0998, 16.3294) -> (-8.8638, 16.3294)
  line L132 (-8.8638, 16.3294) -> (-8.8638, 18.0692)
  line L133 (-8.8638, 18.0692) -> (-11.0998, 18.0692)
  line L134 (-11.0998, 18.0692) -> (-11.0998, 16.3294)
  line L135 (-8.7916, 24.5889) -> (-4.8695, 24.5889)
  line L136 (-5.7125, 23.7458) -> (-7.9485, 23.7458)
  line L137 (-7.9485, 22.0061) -> (-5.7125, 22.0061)
  line L138 (-5.7125, 22.0061) -> (-5.7125, 23.7458)
  line L139 (-7.9485, 23.7458) -> (-7.9485, 22.0061)
  line L140 (-8.7916, 21.163) -> (-8.7916, 24.5889)
  line L141 (-4.8695, 24.5889) -> (-4.8695, 21.163)
  line L142 (-14.8783, 24.5658) -> (-10.9562, 24.5658)
  line L143 (-11.7992, 23.7228) -> (-14.0353, 23.7228)
  line L144 (-14.0353, 21.983) -> (-11.7992, 21.983)
  line L145 (-11.7992, 21.983) -> (-11.7992, 23.7228)
  line L146 (-14.0353, 23.7228) -> (-14.0353, 21.983)
  line L147 (-14.8783, 21.14) -> (-14.8783, 24.5658)
  line L148 (-10.9562, 24.5658) -> (-10.9562, 21.14)
  line L149 (-14.7568, 19.6402) -> (-14.7568, 20.3682)
  line L150 (-4.33, 20.3682) -> (-4.33, 19.6402)
  line L151 (-10.4155, 18.9122) -> (-10.4155, 19.6402)
  line L152 (-9.5321, 19.6402) -> (-9.5321, 18.9122)
  line L153 (-11.9428, 18.9122) -> (-10.4155, 18.9122)
  line L154 (-9.5321, 18.9122) -> (-8.0208, 18.9122)
  line L155 (-4.33, 19.6402) -> (-9.5321, 19.6402)
  line L156 (-10.4155, 19.6402) -> (-14.7568, 19.6402)
  line L157 (-7.3479, 20.3682) -> (-7.3479, 21.163)
  line L158 (-6.5355, 21.163) -> (-6.5355, 20.3682)
  line L159 (-13.5173, 20.3682) -> (-13.5173, 21.14)
  line L160 (-12.5862, 21.14) -> (-12.5862, 20.3682)
  line L161 (-4.8695, 21.163) -> (-6.5355, 21.163)
  line L162 (-7.3479, 21.163) -> (-8.7916, 21.163)
  line L163 (-6.5355, 20.3682) -> (-4.33, 20.3682)
  line L164 (-10.9562, 21.14) -> (-12.5862, 21.14)
  line L165 (-13.5173, 21.14) -> (-14.8783, 21.14)
  line L166 (-14.7568, 20.3682) -> (-13.5173, 20.3682)
  line L167 (-12.5862, 20.3682) -> (-7.3479, 20.3682)
  line L168 (-57.9534, 87.392) -> (-49.5381, 87.392) construction
  line L169 (-49.5381, 87.392) -> (-49.5381, 73.3604) construction
  line L170 (-49.5381, 73.3604) -> (-57.9534, 73.3604) construction
  line L171 (-57.9534, 73.3604) -> (-57.9534, 87.392) construction
  line L172 (-5.5466, 15.8789) -> (-5.5466, 1.508) construction
  line L173 (-5.5466, 1.508) -> (-13.9619, 1.508) construction
  line L174 (-13.9619, 1.508) -> (-13.9619, 15.8789) construction
  line L175 (-13.9619, 15.8789) -> (-5.5466, 15.8789) construction
  line L176 (-1, 12.9669) -> (-1, 1) projected
  line L177 (-31.75, 87.9) -> (-31.75, 1) construction
  line L178 (-62.5, 44.45) -> (-1, 44.45) construction
  line L179 (-93.4198, 68.0127) -> (-88.1904, 68.0127)
  line L180 (-89.3144, 66.8887) -> (-92.2958, 66.8887)
  line L181 (-92.2958, 64.569) -> (-89.3144, 64.569)
  line L182 (-92.2958, 66.8887) -> (-92.2958, 64.569)
  line L183 (-91.4949, 63.445) -> (-93.4198, 63.445)
  line L184 (-93.4198, 63.445) -> (-93.4198, 68.0127)
  line L185 (-88.1904, 68.0127) -> (-88.1904, 63.445)
  line L186 (-88.1904, 63.445) -> (-90.4117, 63.445)
  line L187 (-89.3144, 64.569) -> (-89.3144, 66.8887)
  line L188 (-91.4949, 62.3851) -> (-91.4949, 63.445)
  line L189 (-90.4117, 63.445) -> (-90.4117, 62.3851)
  line L190 (-90.4117, 62.3851) -> (-87.4711, 62.3851)
  line L191 (-87.4711, 62.3851) -> (-87.4711, 61.4145)
  line L192 (-94.4073, 61.4145) -> (-94.4073, 60.4439)
  line L193 (-94.4073, 60.4439) -> (-92.3921, 60.4439)
  line L194 (-87.4711, 61.4145) -> (-94.4073, 61.4145)
  line L195 (-99.7209, 62.3851) -> (-99.7209, 63.4142)
  line L196 (-97.4301, 64.5382) -> (-97.4301, 66.8579)
  line L197 (-95.5851, 61.4145) -> (-101.3735, 61.4145)
  line L198 (-101.3735, 61.4145) -> (-101.3735, 62.3851)
  line L199 (-101.3735, 62.3851) -> (-99.7209, 62.3851)
  line L200 (-100.4114, 64.5382) -> (-97.4301, 64.5382)
  line L201 (-96.306, 67.9819) -> (-96.306, 63.4142)
  line L202 (-100.4114, 66.8579) -> (-100.4114, 64.5382)
  line L203 (-97.4301, 66.8579) -> (-100.4114, 66.8579)
  line L204 (-101.5355, 67.9819) -> (-96.306, 67.9819)
  line L205 (-101.5355, 63.4142) -> (-101.5355, 67.9819)
  line L206 (-99.7209, 63.4142) -> (-101.5355, 63.4142)
  line L207 (-92.3921, 55.8761) -> (-97.6215, 55.8761)
  line L208 (-97.6215, 55.8761) -> (-97.6215, 60.4439)
  line L209 (-92.3921, 60.4439) -> (-92.3921, 55.8761)
  line L210 (-96.4975, 57.0001) -> (-93.5161, 57.0001)
  line L211 (-93.5161, 57.0001) -> (-93.5161, 59.3198)
  line L212 (-93.5161, 59.3198) -> (-96.4975, 59.3198)
  line L213 (-96.4975, 59.3198) -> (-96.4975, 57.0001)
  line L214 (-98.4793, 63.4142) -> (-98.4793, 62.3851)
  line L215 (-96.306, 63.4142) -> (-98.4793, 63.4142)
  line L216 (-95.5851, 60.4439) -> (-95.5851, 61.4145)
  line L217 (-97.6215, 60.4439) -> (-95.5851, 60.4439)
  line L218 (-98.4793, 62.3851) -> (-91.4949, 62.3851)
  line L219 (-24.196, 69.4211) -> (-29.4255, 69.4211)
  line L220 (-28.3014, 70.5451) -> (-25.3201, 70.5451)
  line L221 (-25.3201, 72.8648) -> (-28.3014, 72.8648)
  line L222 (-25.3201, 70.5451) -> (-25.3201, 72.8648)
  line L223 (-26.121, 73.9888) -> (-24.196, 73.9888)
  line L224 (-24.196, 73.9888) -> (-24.196, 69.4211)
  line L225 (-29.4255, 69.4211) -> (-29.4255, 73.9888)
  line L226 (-29.4255, 73.9888) -> (-27.2041, 73.9888)
  line L227 (-28.3014, 72.8648) -> (-28.3014, 70.5451)
  line L228 (-26.121, 75.0487) -> (-26.121, 73.9888)
  line L229 (-27.2041, 73.9888) -> (-27.2041, 75.0487)
  line L230 (-27.2041, 75.0487) -> (-30.1447, 75.0487)
  line L231 (-30.1447, 75.0487) -> (-30.1447, 76.0192)
  line L232 (-23.2086, 76.0192) -> (-23.2086, 76.9899)
  line L233 (-23.2086, 76.9899) -> (-25.2237, 76.9899)
  line L234 (-30.1447, 76.0192) -> (-23.2086, 76.0192)
  line L235 (-17.895, 75.0487) -> (-17.895, 74.0196)
  line L236 (-20.1858, 72.8956) -> (-20.1858, 70.5759)
  line L237 (-22.0307, 76.0192) -> (-16.2423, 76.0192)
  line L238 (-16.2423, 76.0192) -> (-16.2423, 75.0487)
  line L239 (-16.2423, 75.0487) -> (-17.895, 75.0487)
  line L240 (-17.2044, 72.8956) -> (-20.1858, 72.8956)
  line L241 (-21.3098, 69.4518) -> (-21.3098, 74.0196)
  line L242 (-17.2044, 70.5759) -> (-17.2044, 72.8956)
  line L243 (-20.1858, 70.5759) -> (-17.2044, 70.5759)
  line L244 (-16.0804, 69.4518) -> (-21.3098, 69.4518)
  line L245 (-16.0804, 74.0196) -> (-16.0804, 69.4518)
  line L246 (-17.895, 74.0196) -> (-16.0804, 74.0196)
  line L247 (-25.2237, 81.5577) -> (-19.9943, 81.5577)
  line L248 (-19.9943, 81.5577) -> (-19.9943, 76.9899)
  line L249 (-25.2237, 76.9899) -> (-25.2237, 81.5577)
  line L250 (-21.1183, 80.4336) -> (-24.0997, 80.4336)
  line L251 (-24.0997, 80.4336) -> (-24.0997, 78.114)
  line L252 (-24.0997, 78.114) -> (-21.1183, 78.114)
  line L253 (-21.1183, 78.114) -> (-21.1183, 80.4336)
  line L254 (-19.1365, 74.0196) -> (-19.1365, 75.0487)
  line L255 (-21.3098, 74.0196) -> (-19.1365, 74.0196)
  line L256 (-22.0307, 76.9899) -> (-22.0307, 76.0192)
  line L257 (-19.9943, 76.9899) -> (-22.0307, 76.9899)
  line L258 (-19.1365, 75.0487) -> (-26.121, 75.0487)
  line L259 (-43.3142, 16.0044) -> (-43.3142, 18.3241)
  line L260 (-39.304, 19.4789) -> (-34.0745, 19.4789)
  line L261 (-35.1986, 18.3549) -> (-38.1799, 18.3549)
  line L262 (-38.1799, 18.3549) -> (-38.1799, 16.0352)
  line L263 (-41.4693, 12.8808) -> (-47.2577, 12.8808)
  line L264 (-37.379, 14.9112) -> (-39.304, 14.9112)
  line L265 (-38.1799, 16.0352) -> (-35.1986, 16.0352)
  line L266 (-33.3553, 12.8808) -> (-40.2914, 12.8808)
  line L267 (-37.379, 13.8513) -> (-37.379, 14.9112)
  line L268 (-36.2959, 14.9112) -> (-36.2959, 13.8513)
  line L269 (-34.0745, 14.9112) -> (-36.2959, 14.9112)
  line L270 (-36.2959, 13.8513) -> (-33.3553, 13.8513)
  line L271 (-35.1986, 16.0352) -> (-35.1986, 18.3549)
  line L272 (-34.0745, 19.4789) -> (-34.0745, 14.9112)
  line L273 (-45.605, 13.8513) -> (-45.605, 14.8804)
  line L274 (-40.2914, 12.8808) -> (-40.2914, 11.9101)
  line L275 (-39.304, 14.9112) -> (-39.304, 19.4789)
  line L276 (-40.2914, 11.9101) -> (-38.2763, 11.9101)
  line L277 (-33.3553, 13.8513) -> (-33.3553, 12.8808)
  line L278 (-42.1902, 19.4482) -> (-42.1902, 14.8804)
  line L279 (-46.2956, 18.3241) -> (-46.2956, 16.0044)
  line L280 (-46.2956, 16.0044) -> (-43.3142, 16.0044)
  line L281 (-43.3142, 18.3241) -> (-46.2956, 18.3241)
  line L282 (-47.4196, 19.4482) -> (-42.1902, 19.4482)
  line L283 (-47.2577, 13.8513) -> (-45.605, 13.8513)
  line L284 (-47.2577, 12.8808) -> (-47.2577, 13.8513)
  line L285 (-47.4196, 14.8804) -> (-47.4196, 19.4482)
  line L286 (-44.3635, 13.8513) -> (-37.379, 13.8513)
  line L287 (-41.4693, 11.9101) -> (-41.4693, 12.8808)
  line L288 (-43.5057, 11.9101) -> (-41.4693, 11.9101)
  line L289 (-42.3817, 10.786) -> (-42.3817, 8.4664)
  line L290 (-39.4003, 8.4664) -> (-39.4003, 10.786)
  line L291 (-42.3817, 8.4664) -> (-39.4003, 8.4664)
  line L292 (-39.4003, 10.786) -> (-42.3817, 10.786)
  line L293 (-44.3635, 14.8804) -> (-44.3635, 13.8513)
  line L294 (-42.1902, 14.8804) -> (-44.3635, 14.8804)
  line L295 (-38.2763, 11.9101) -> (-38.2763, 7.3423)
  line L296 (-38.2763, 7.3423) -> (-43.5057, 7.3423)
  line L297 (-43.5057, 7.3423) -> (-43.5057, 11.9101)
  line L298 (-45.605, 14.8804) -> (-47.4196, 14.8804)
  line L299 (-25.6449, 16.0044) -> (-25.6449, 18.3241)
  line L300 (-21.6347, 19.4789) -> (-16.4052, 19.4789)
  line L301 (-17.5293, 18.3549) -> (-20.5106, 18.3549)
  line L302 (-20.5106, 18.3549) -> (-20.5106, 16.0352)
  line L303 (-23.8, 12.8808) -> (-29.5884, 12.8808)
  line L304 (-19.7097, 14.9112) -> (-21.6347, 14.9112)
  line L305 (-20.5106, 16.0352) -> (-17.5293, 16.0352)
  line L306 (-15.686, 12.8808) -> (-22.6221, 12.8808)
  line L307 (-19.7097, 13.8513) -> (-19.7097, 14.9112)
  line L308 (-18.6266, 14.9112) -> (-18.6266, 13.8513)
  line L309 (-16.4052, 14.9112) -> (-18.6266, 14.9112)
  line L310 (-18.6266, 13.8513) -> (-15.686, 13.8513)
  line L311 (-17.5293, 16.0352) -> (-17.5293, 18.3549)
  line L312 (-16.4052, 19.4789) -> (-16.4052, 14.9112)
  line L313 (-27.9357, 13.8513) -> (-27.9357, 14.8804)
  line L314 (-22.6221, 12.8808) -> (-22.6221, 11.9101)
  line L315 (-21.6347, 14.9112) -> (-21.6347, 19.4789)
  line L316 (-22.6221, 11.9101) -> (-20.607, 11.9101)
  line L317 (-15.686, 13.8513) -> (-15.686, 12.8808)
  line L318 (-24.5209, 19.4482) -> (-24.5209, 14.8804)